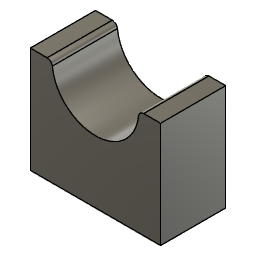
PVC Support v1 (Autodesk Fusion 360 design; units mm, degrees)
Autodesk Fusion 360 part; units mm, degrees
sketch "Sketch1" plane through (0, 0, 0) normal (0, 0, 1) x (1, 0, 0)
  line L0 (50, 40.65) -> (50, 0)
  line L1 (50, 0) -> (0, 0)
  line L2 (0, 0) -> (0, 40.65)
  line L3 (6.4575, 40.65) -> (0, 40.65)
  line L4 (43.5425, 40.65) -> (50, 40.65)
  arc A0 (8.446, 38.8645) -> (41.554, 38.8645) centre (25, 40.65) ccw
  arc A1 (8.446, 38.8645) -> (6.4575, 40.65) centre (6.4575, 38.65) ccw
  arc A2 (43.5425, 40.65) -> (41.554, 38.8645) centre (43.5425, 38.65) ccw
  dimension "d1" = 33.3
  dimension "d2" = 40.65
  dimension "d3" = 2
  constraint vertical L0
  constraint horizontal L1
  constraint vertical L2
  constraint perpendicular L2 L3
  constraint perpendicular L0 L4
  constraint tangent A0 A1
  constraint tangent L3 A1
  constraint tangent A0 A2
  constraint tangent L4 A2
  constraint equal A1 A2
  measures "d1" diameter of A0
  measures "d2" distance of L1 A0.centre
  measures "d3" radius of A1
extrude "Extrude1" add sketch "Sketch1" against normal blind 25
